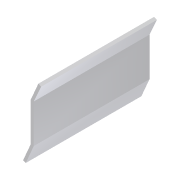
# Autodesk Inventor part: PChook
Saved by Autodesk Inventor 2015 (Build 190159000, 159)
## iProperties
Created: 2015-03-07
Part Number: PChook
Material: Polycarbonate, Clear
Document SubType Name: Modeling
Designer: Jaden
Density: 1.2 g/cm^3
Appearance: Polycarbonate - Clear
Author: Jaden
Autodesk Inventor part; units mm, degrees
ref_plane "YZ Plane" through (0, 0, 0) normal (1, 0, 0) x (0, 1, 0)
ref_plane "XZ Plane" through (0, 0, 0) normal (0, 1, 0) x (-1, 0, 0)
ref_plane "XY Plane" through (0, 0, 0) normal (0, 0, 1) x (1, 0, 0)
sketch "Sketch1" plane through (0, 0, 0) normal (0, 0, 1) x (1, 0, 0)
  line L0 (0, 0) -> (5.0316, 11.6608)
  line L1 (0, 0) -> (12.7, 0) construction
  line L2 (5.0316, 11.6608) -> (5.0316, 37.0608)
  line L3 (5.0316, 37.0608) -> (10.0631, 48.7215)
  line L4 (10.0631, 48.7215) -> (11.9289, 47.9165)
  line L5 (7.0636, 37.0608) -> (11.9289, 47.9165)
  line L6 (7.0636, 37.0608) -> (7.0636, 11.6608)
  line L7 (7.0636, 11.6608) -> (1.713, -0.7392)
  line L8 (1.713, -0.7392) -> (0, 0)
  dimension "d8" = 12.7
  dimension "d9" = 66.66
  dimension "d11" = 12.7
  dimension "d12" = 156.66
  dimension "d13" = 2.032
  dimension "d14" = 2.032
  constraints: 18 end point, 2 perpendicular, 2 vertical, 1 equal length, 1 horizontal, 1 parallel
  measures "d8" distance of L0.start L0.end
  measures "d9" angle of L1 L0
  measures "d11" distance of L2.end L3.end
  measures "d12" angle of L2 L3
  measures "d13" distance of L3.end L4.end
  measures "d14" distance of L2.end L5.start
extrude "Extrusion1" add sketch "Sketch1" along normal blind 76.2
body "Solid1"
